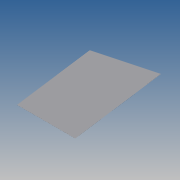
# Autodesk Inventor part: panelEflat
Saved by Autodesk Inventor 2014 SP1 (Build 180222100, 222)
## iProperties
Created: 2015-02-13
Part Number: panelEflat
Material: Generic
Document SubType Name: Modeling
Designer: Dave
Density: 1 g/cm^3
Appearance: Default
Author: Dave
Autodesk Inventor part; units mm, degrees
ref_plane "YZ Plane" through (0, 0, 0) normal (1, 0, 0) x (0, 1, 0)
ref_plane "XZ Plane" through (0, 0, 0) normal (0, 1, 0) x (-1, 0, 0)
ref_plane "XY Plane" through (0, 0, 0) normal (0, 0, 1) x (1, 0, 0)
sketch "Sketch1" plane through (0, 0, 0) normal (0, 1, 0) x (-1, 0, 0)
  line L0 (0, 0) -> (-8000, 0) construction
  line L1 (0, 0) -> (-7727.4066, -2070.5524) construction
  line L2 (0, 0) -> (8000, 0) construction
  line L3 (0, 0) -> (-6335.3327, -834.0624) construction
  line L4 (0, 0) -> (6390, 0) construction
  line L5 (-7681.4421, 50) -> (-7406.7624, -2036.3998)
  line L6 (-6218.9436, -1718.1247) -> (-6451.7217, 50)
  line L7 (-6218.9436, -1718.1247) -> (-7406.7624, -2036.3998)
  line L8 (-6451.7217, 50) -> (-7681.4421, 50)
  dimension "d0" = 8000
  dimension "d1" = 8000
  dimension "d2" = 165
  dimension "d3" = 6390
  dimension "d4" = 172.5
  dimension "d7" = 50
  dimension "d8" = 50
  constraints: 18 end point, 3 horizontal, 3 parallel, 2 equal length, 1 midpoint
  measures "d0" distance of L0.start L0.end
  measures "d1" distance of L0.start L1.end
  measures "d2" angle of L1 L2
  measures "d3" distance of L3.end L0.start
  measures "d4" angle of L3 L4
  measures "d7" distance between parallel lines of L1 L7
  measures "d8" distance between parallel lines of L8 L0
extrude "Extrusion1" add sketch "Sketch1" along normal blind 1
body "Solid1"
